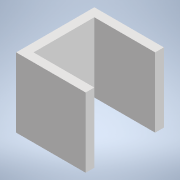
# Autodesk Inventor part: connector
Saved by Autodesk Inventor 2020.2 (Build 242310000, 310)
## iProperties
Created: 2020-03-20
Part Number: connector
Material: Generic
Document SubType Name: Modeling
Designer: deli
Density: 1 g/cm^3
Appearance: Default
Author: deli
Autodesk Inventor part; units mm, degrees
ref_plane "YZ Plane" through (0, 0, 0) normal (1, 0, 0) x (0, 1, 0)
ref_plane "XZ Plane" through (0, 0, 0) normal (0, 1, 0) x (-1, 0, 0)
ref_plane "XY Plane" through (0, 0, 0) normal (0, 0, 1) x (1, 0, 0)
sketch "Sketch1" plane through (0, 0, 0) normal (0, 1, 0) x (-1, 0, 0)
  line L0 (22.3541, -3128.9614) -> (-9.3959, -3128.9614)
  line L1 (-9.3959, -3128.9614) -> (-9.3959, -3132.1364)
  line L2 (-9.3959, -3132.1364) -> (22.3541, -3132.1364)
  line L3 (22.3541, -3132.1364) -> (22.3541, -3128.9614)
  line L4 (22.3541, -3128.9614) -> (19.1791, -3128.9614)
  line L5 (19.1791, -3128.9614) -> (19.1791, -3157.5364)
  line L6 (19.1791, -3157.5364) -> (22.3541, -3157.5364)
  line L7 (22.3541, -3157.5364) -> (22.3541, -3128.9614)
  line L8 (22.3541, -3157.5364) -> (-9.3959, -3157.5364)
  line L9 (-9.3959, -3157.5364) -> (-9.3959, -3160.7114)
  line L10 (-9.3959, -3160.7114) -> (22.3541, -3160.7114)
  line L11 (22.3541, -3160.7114) -> (22.3541, -3157.5364)
  point P0 (0, 0)
  point P1 (19.1791, -3132.1364)
  dimension "d0" = 31.75
  dimension "d1" = 3.175
  dimension "d2" = 3.175
  dimension "d4" = 31.75
  dimension "d5" = 3.175
  dimension "d22" = 31.75
  constraints: 24 end point, 6 parallel, 3 horizontal, 3 perpendicular
  measures "d0" distance of L2.end L1.end
  measures "d1" distance of L1.end L0.end
  measures "d2" distance of L6.end L5.end
  measures "d4" distance of L10.end L9.end
  measures "d5" distance of L9.end L8.end
  measures "d22" distance between parallel lines of L0 L10
extrude "Extrusion1" add sketch "Sketch1" along normal blind 22.225
sketch "Sketch2" plane through (-19.1791, 0, -3132.1364) normal (1, 0, 0) x (0, 0, -1)
  line L0 (-3.175, 0) -> (0, 0) projected
  line L1 (0, 0) -> (0, 22.225) projected
  line L2 (-3.175, 22.225) -> (0, 22.225) projected
  line L3 (-3.175, 0) -> (-3.175, 22.225) projected
  line L4 (25.4, 0) -> (28.575, 0) projected
  line L5 (28.575, 0) -> (28.575, 22.225) projected
  line L6 (25.4, 22.225) -> (28.575, 22.225) projected
  line L7 (25.4, 0) -> (25.4, 22.225) projected
  circle A0 centre (5.08, 17.145) radius 1.8542
  circle A1 centre (20.32, 17.145) radius 1.8542
  circle A2 centre (5.08, 5.08) radius 1.8542
  circle A3 centre (20.32, 5.08) radius 1.8542
  line L8 (0, 22.225) -> (25.4, 22.225) projected
  line L9 (0, 0) -> (25.4, 0) projected
  point P0 (-3132.1364, 0)
  dimension "d8" = 3.7084
  dimension "d9" = 3.7084
  dimension "d10" = 3.7084
  dimension "d11" = 3.7084
  dimension "d12" = 5.08
  dimension "d13" = 5.08
  dimension "d14" = 5.08
  dimension "d15" = 5.08
  dimension "d16" = 5.08
  dimension "d17" = 5.08
  dimension "d18" = 5.08
  dimension "d19" = 5.08
  constraints: 4 centre point
  measures "d8" diameter of A0
  measures "d9" diameter of A1
  measures "d10" diameter of A2
  measures "d11" diameter of A3
  measures "d12" distance from line of L7 A3.centre
  measures "d13" distance from line of L1 A2.centre
  measures "d14" distance from line of L1 A0.centre
  measures "d15" distance from line of L7 A1.centre
  measures "d16" distance from line of L8 A0.centre
  measures "d17" distance from line of L8 A1.centre
  measures "d18" distance from line of L9 A3.centre
  measures "d19" distance from line of L9 A2.centre
extrude "Extrusion2" cut sketch "Sketch2" against normal blind 25.4 contours A0 | A1 | A2 | A3
sketch "Sketch3" plane through (-22.3541, 0, -3128.9614) normal (0, 0, 1) x (1, 0, 0)
  circle A0 centre (26.67, 17.145) radius 1.8542
  circle A1 centre (11.43, 17.145) radius 1.8542
  circle A2 centre (26.67, 5.08) radius 1.8542
  circle A3 centre (11.43, 5.08) radius 1.8542
  line L0 (0, 0) -> (31.75, 0) projected
  line L1 (31.75, 0) -> (31.75, 22.225) projected
  line L2 (0, 22.225) -> (31.75, 22.225) projected
  line L3 (0, 0) -> (0, 22.225) projected
  point P0 (22.3541, 0)
  dimension "d23" = 3.7084
  dimension "d24" = 3.7084
  dimension "d25" = 3.7084
  dimension "d26" = 3.7084
  dimension "d27" = 5.08
  dimension "d28" = 5.08
  dimension "d29" = 11.43
  dimension "d30" = 11.43
  dimension "d31" = 5.08
  dimension "d32" = 5.08
  dimension "d33" = 5.08
  dimension "d34" = 5.08
  constraints: 4 centre point
  measures "d23" diameter of A0
  measures "d24" diameter of A1
  measures "d25" diameter of A2
  measures "d26" diameter of A3
  measures "d27" distance from line of L1 A0.centre
  measures "d28" distance from line of L1 A2.centre
  measures "d29" distance from line of L3 A3.centre
  measures "d30" distance from line of L3 A1.centre
  measures "d31" distance from line of L2 A1.centre
  measures "d32" distance from line of L2 A0.centre
  measures "d33" distance from line of L0 A2.centre
  measures "d34" distance from line of L0 A3.centre
extrude "Extrusion3" cut sketch "Sketch3" against normal blind 50.8 contours A0 | A1 | A2 | A3
equation "\"d4\" = d0"
equation "\"d13\" = d12"
equation "\"d14\" = d12"
equation "\"d15\" = d12"
equation "\"d17\" = d16"
equation "\"d18\" = d16"
equation "\"d19\" = d16"
equation "\"d28\" = d27"
equation "\"d30\" = d29"
equation "\"d32\" = d31"
equation "\"d33\" = d31"
equation "\"d34\" = d31"
body "Solid1"
